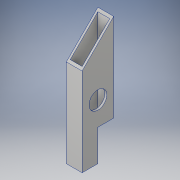
# Autodesk Inventor part: BottomStorageSupport.ver1-1111-2020
Saved by Autodesk Inventor 2018 (Build 220112000, 112)
## iProperties
Created: 2020-01-20
Part Number: BottomStorageSupport.ver1-1111-2020
Material: Aluminum 6061
Document SubType Name: Modeling
Designer: JMHal
Density: 2.7 g/cm^3
Appearance: Aluminum - Flat
Author: JMHal
Autodesk Inventor part; units mm, degrees
ref_plane "YZ Plane" through (0, 0, 0) normal (1, 0, 0) x (0, 1, 0)
ref_plane "XZ Plane" through (0, 0, 0) normal (0, 1, 0) x (-1, 0, 0)
ref_plane "XY Plane" through (0, 0, 0) normal (0, 0, 1) x (1, 0, 0)
sketch "Sketch1" plane through (0, 0, 0) normal (0, 1, 0) x (-1, 0, 0)
  line L0 (0, 0) -> (25.4, 0)
  line L1 (25.4, 0) -> (25.4, -25.4)
  line L2 (25.4, -25.4) -> (0, -25.4)
  line L3 (0, -25.4) -> (0, 0)
  line L4 (22.225, -22.225) -> (22.225, -3.175)
  line L5 (22.225, -3.175) -> (3.175, -3.175)
  line L6 (3.175, -3.175) -> (3.175, -22.225)
  line L7 (3.175, -22.225) -> (22.225, -22.225)
  dimension "d0" = 25.4
  dimension "d1" = 25.4
  dimension "d2" = 3.175
  constraints: 16 end point, 4 parallel, 2 perpendicular, 1 horizontal, 3 other
  measures "d0" distance of L1.end L2.end
  measures "d1" distance of L0.end L1.end
  measures "d2" distance between parallel lines of L1 L4
extrude "Extrusion1" add sketch "Sketch1" along normal blind 141.7828
sketch "Sketch2" plane through (0, 0, 0) normal (1, 0, 0) x (0, 0, -1)
  line L0 (25.4, 0) -> (0, 0) projected
  line L1 (25.4, 0) -> (25.4, 141.7828) projected
  line L2 (0, 141.7828) -> (25.4, 141.7828) projected
  line L3 (0, 0) -> (0, 141.7828) projected
  line L4 (0, 141.7828) -> (25.4, 141.7828)
  line L5 (25.4, 141.7828) -> (25.4, 116.3828)
  line L6 (25.4, 116.3828) -> (0, 116.3828)
  line L7 (0, 116.3828) -> (0, 141.7828)
  line L8 (25.4, 0) -> (25.4, 141.7828) projected
  line L9 (25.4, 141.7828) -> (0, 116.3828)
  dimension "d5" = 45
  constraints: 10 end point, 2 parallel, 1 horizontal, 1 perpendicular, 1 point on line
  measures "d5" angle of L3 L9
extrude "Extrusion2" cut sketch "Sketch2" against normal blind 141.7828 contours L3 L2 L9
sketch "Sketch3" plane through (0, 0, 0) normal (0, -1, 0) x (1, 0, 0)
  line L0 (-3.175, -22.225) -> (-22.225, -22.225) projected
  line L1 (-22.225, -22.225) -> (-22.225, -3.175) projected
  line L2 (-22.225, -3.175) -> (-3.175, -3.175) projected
  line L3 (-3.175, -3.175) -> (-3.175, -22.225) projected
  line L4 (0, 0) -> (-25.4, 0) projected
  line L5 (-25.4, 0) -> (-25.4, -25.4) projected
  line L6 (-25.4, -25.4) -> (0, -25.4) projected
  line L7 (0, -25.4) -> (0, 0) projected
  line L8 (0, 0) -> (-25.4, 0)
  line L9 (-25.4, 0) -> (-25.4, 25.4)
  line L10 (-25.4, 25.4) -> (0, 25.4)
  line L11 (0, 25.4) -> (0, 0)
  line L12 (-3.175, -3.175) -> (-22.225, -3.175)
  line L13 (-22.225, -3.175) -> (-22.225, 22.225)
  line L14 (-22.225, 22.225) -> (-3.175, 22.225)
  line L15 (-3.175, 22.225) -> (-3.175, -3.175)
  line L16 (-3.175, 22.225) -> (-22.225, 22.225)
  line L17 (-22.225, 22.225) -> (-22.225, 0)
  line L18 (-22.225, 0) -> (-3.175, 0)
  line L19 (-3.175, 0) -> (-3.175, 22.225)
  line L20 (-3.175, 0) -> (-22.225, 0)
  line L21 (-22.225, 0) -> (-22.225, -3.175)
  line L22 (-22.225, -3.175) -> (-3.175, -3.175)
  line L23 (-3.175, -3.175) -> (-3.175, 0)
  line L24 (0, 25.4) -> (-25.4, 25.4)
  line L25 (-25.4, 25.4) -> (-25.4, 0)
  line L26 (-25.4, 0) -> (0, 0)
  line L27 (0, 0) -> (0, 25.4)
  dimension "d8" = 25.4
  dimension "d9" = 25.4
  dimension "d10" = 19.05
  dimension "d11" = 3.175
  constraints: 40 end point, 10 parallel, 5 horizontal, 5 perpendicular, 2 point on line
  measures "d8" distance of L9.end L10.end
  measures "d9" distance of L8.end L9.end
  measures "d10" distance of L13.end L14.end
  measures "d11" distance between parallel lines of L10 L14
extrude "Extrusion3" add sketch "Sketch3" against normal blind 127 contours L15 L14 L13 L4 L9 L10 L11
extrude "Extrusion4" cut sketch "Sketch3" against normal through all contours L2 L13 L4 L15
sketch "Sketch4" plane through (0, 0, -25.4) normal (1, 0, 0) x (0, 0, -1)
  line L0 (0, 141.7828) -> (-25.4, 116.3828) projected
  line L1 (-25.4, 116.3828) -> (-25.4, 127) projected
  line L2 (-50.8, 127) -> (-25.4, 127) projected
  line L3 (-50.8, 0) -> (-50.8, 127) projected
  line L4 (0, 0) -> (-50.8, 0) projected
  line L5 (0, 0) -> (0, 141.7828) projected
  line L6 (-25.4, 116.3828) -> (-50.8, 90.9828)
  line L7 (-50.8, 0) -> (-50.8, 127) projected
  point P0 (-25.4, 0)
  constraints: 2 end point, 1 point on line
extrude "Extrusion5" cut sketch "Sketch4" against normal blind 127 contours L6 L3 L2 L1
sketch "Sketch5" plane through (0, 0, 0) normal (0, -1, 0) x (1, 0, 0)
  line L0 (-3.175, 22.225) -> (-3.175, -22.225) projected
  line L1 (-3.175, -22.225) -> (-22.225, -22.225) projected
  line L2 (-22.225, -22.225) -> (-22.225, 22.225) projected
  line L3 (-22.225, 22.225) -> (-3.175, 22.225) projected
  line L4 (-25.4, 25.4) -> (-25.4, -25.4) projected
  line L5 (-25.4, -25.4) -> (0, -25.4) projected
  line L6 (0, -25.4) -> (0, 25.4) projected
  line L7 (0, 25.4) -> (-25.4, 25.4) projected
  line L8 (0, 25.4) -> (-25.4, 25.4)
  line L9 (-25.4, 25.4) -> (-25.4, 0)
  line L10 (-25.4, 0) -> (0, 0)
  line L11 (0, 0) -> (0, 25.4)
  line L12 (-3.175, 22.225) -> (-3.175, -22.225) projected
  line L13 (-22.225, 22.225) -> (-3.175, 22.225) projected
  line L14 (-3.175, 0) -> (-3.175, 22.225)
  line L15 (-3.175, 22.225) -> (-22.225, 22.225)
  line L16 (-22.225, 22.225) -> (-22.225, 0)
  line L17 (-22.225, -22.225) -> (-22.225, 22.225) projected
  line L18 (-3.175, 22.225) -> (-22.225, 22.225)
  line L19 (-22.225, 22.225) -> (-22.225, 0)
  line L20 (-22.225, 0) -> (-3.175, 0)
  line L21 (-3.175, 0) -> (-3.175, 22.225)
  line L22 (0, 25.4) -> (-25.4, 25.4)
  line L23 (-25.4, 25.4) -> (-25.4, 0)
  line L24 (-25.4, 0) -> (0, 0)
  line L25 (0, 0) -> (0, 25.4)
  constraints: 30 end point, 7 equal length, 4 perpendicular, 3 horizontal, 3 midpoint
extrude "Extrusion6" add sketch "Sketch5" along normal blind 50.8 contours L3 L2 L10 L4 L7 L6 L0
sketch "Sketch6" plane through (0, 0, -25.4) normal (1, 0, 0) x (0, 0, -1)
  line L0 (0, 141.7828) -> (-50.8, 90.9828) projected
  line L1 (-50.8, -50.8) -> (-50.8, 90.9828) projected
  line L2 (-25.4, -50.8) -> (-50.8, -50.8) projected
  line L3 (-25.4, 0) -> (-25.4, -50.8) projected
  line L4 (0, 0) -> (-25.4, 0) projected
  line L5 (0, 0) -> (0, 141.7828) projected
  point P0 (-25.4, 38.1)
  dimension "d20" = 38.1
  dimension "d21" = 25.4
  measures "d20" distance from line of point (-25.4, 38.1) L4
  measures "d21" distance from line of L5 point (-25.4, 38.1)
hole "Hole1" at (0, 38.1, 0) direction (-1, 0, 0) diameter 28.575 end through all
body "Solid1"
